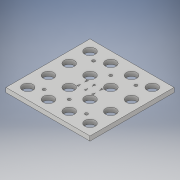
# Autodesk Inventor part: back_plate
Saved by Autodesk Inventor 2019 (Build 230136000, 136)
## iProperties
Created: 2019-08-25
Part Number: back_plate
Material: Generic
Document SubType Name: Modeling
Designer: Lino P
Density: 1 g/cm^3
Appearance: Default
Author: Lino P
Autodesk Inventor part; units mm, degrees
ref_plane "YZ Plane" through (0, 0, 0) normal (1, 0, 0) x (0, 1, 0)
ref_plane "XZ Plane" through (0, 0, 0) normal (0, 1, 0) x (-1, 0, 0)
ref_plane "XY Plane" through (0, 0, 0) normal (0, 0, 1) x (1, 0, 0)
sketch "Sketch1" plane through (0, 0, 0) normal (0, 1, 0) x (-1, 0, 0)
  line L0 (-85, 85) -> (85, 85)
  line L1 (85, 85) -> (85, -85)
  line L2 (85, -85) -> (-85, -85)
  line L3 (-85, -85) -> (-85, 85)
  line L4 (-85, 85) -> (85, -85) construction
  line L5 (85, 85) -> (-85, -85) construction
  point P0 (0, 0)
  point P1 (-63, -63)
  point P2 (-63, -21)
  point P3 (-63, 21)
  point P4 (-63, 63)
  point P5 (-21, -63)
  point P6 (-21, -21)
  point P7 (-21, 21)
  point P8 (-21, 63)
  point P9 (21, -63)
  point P10 (21, -21)
  point P11 (21, 21)
  point P12 (21, 63)
  point P13 (63, -63)
  point P14 (63, -21)
  point P15 (63, 21)
  point P16 (63, 63)
  dimension "d0" = 170
  dimension "d1" = 170
  dimension "d4" = 42
  dimension "d7" = 42
  constraints: 12 end point, 2 horizontal, 2 midpoint, 2 parallel, 1 perpendicular, 1 vertical, 15 other
  measures "d0" distance of L1.end L2.end
  measures "d1" distance of L0.end L1.end
  measures "d4" distance of point (-63, -63) point (-63, -21)
  measures "d7" distance of point (-63, -63) point (-21, -63)
extrude "Extrusion1" add sketch "Sketch1" along normal blind 9
hole "Hole1" at (63, 0, -63) at (63, 0, -21) at (63, 0, 21) at (63, 0, 63) at (21, 0, -63) at (21, 0, -21) at (21, 0, 21) at (21, 0, 63) at (-21, 0, -63) at (-21, 0, -21) at (-21, 0, 21) at (-21, 0, 63) at (-63, 0, -63) at (-63, 0, -21) at (-63, 0, 21) at (-63, 0, 63) direction (0, 1, 0) diameter 21 end through all both
sketch "Sketch2" plane through (0, 9, 0) normal (0, 1, 0) x (1, 0, 0)
  line L0 (-33.7, -4.15) -> (33.7, -4.15)
  line L1 (33.7, -4.15) -> (33.7, 4.15)
  line L2 (33.7, 4.15) -> (-33.7, 4.15)
  line L3 (-33.7, 4.15) -> (-33.7, -4.15)
  line L4 (-33.7, -4.15) -> (33.7, 4.15) construction
  line L5 (33.7, -4.15) -> (-33.7, 4.15) construction
  point P0 (0, 0)
  dimension "d19" = 67.4
  dimension "d20" = 8.3
  constraints: 12 end point, 2 midpoint, 2 parallel, 1 horizontal, 1 perpendicular
  measures "d19" distance of L2.end L1.end
  measures "d20" distance of L1.end L0.end
sketch "Sketch3" plane through (0, 9, 0) normal (0, 1, 0) x (1, 0, 0)
  line L0 (-42.7949, -50) -> (42.7949, -50) construction
  line L1 (42.7949, -50) -> (42.7949, 50) construction
  line L2 (42.7949, 50) -> (-42.7949, 50) construction
  line L3 (-42.7949, 50) -> (-42.7949, -50) construction
  line L4 (-42.7949, -50) -> (42.7949, 50) construction
  line L5 (42.7949, -50) -> (-42.7949, 50) construction
  point P0 (25, -42.5)
  point P1 (0, 0)
  dimension "d31" = 100
  constraints: 12 end point, 4 coincident, 2 midpoint, 2 parallel, 1 horizontal, 1 perpendicular
  measures "d31" distance of L1.end L0.end
hole "Hole3" at (-42.7949, 9, -50) at (42.7949, 9, -50) at (42.7949, 9, 50) at (-42.7949, 9, 50) direction (0, -1, 0) diameter 6 end through all both
sketch "Sketch4" plane through (0, 9, 0) normal (0, 1, 0) x (1, 0, 0)
  circle A0 centre (42.7949, -50) radius 3 construction
  circle A1 centre (-42.7949, 50) radius 3 construction
  circle A2 centre (42.7949, 50) radius 3 construction
  circle A3 centre (-42.7949, -50) radius 3 construction
  circle A4 centre (-63, -21) radius 10.5 construction
  circle A5 centre (-63, 63) radius 10.5 construction
  circle A6 centre (-21, -21) radius 10.5 construction
  circle A7 centre (-21, 63) radius 10.5 construction
  circle A8 centre (21, -21) radius 10.5 construction
  circle A9 centre (21, 63) radius 10.5 construction
  circle A10 centre (63, -21) radius 10.5 construction
  circle A11 centre (63, 63) radius 10.5 construction
  circle A12 centre (63, 21) radius 10.5 construction
  circle A13 centre (63, -63) radius 10.5 construction
  circle A14 centre (21, 21) radius 10.5 construction
  circle A15 centre (21, -63) radius 10.5 construction
  circle A16 centre (-21, 21) radius 10.5 construction
  circle A17 centre (-21, -63) radius 10.5 construction
  circle A18 centre (-63, 21) radius 10.5 construction
  circle A19 centre (-63, -63) radius 10.5 construction
  line L0 (-85, -85) -> (85, -85) construction
  line L1 (85, -85) -> (85, 85) construction
  line L2 (85, 85) -> (-85, 85) construction
  line L3 (-85, 85) -> (-85, -85) construction
  line L4 (-85, 85) -> (85, 85) construction
  line L5 (-7.5, -85) -> (7.5, -85) construction
  line L6 (7.5, -85) -> (7.5, 85) construction
  line L7 (7.5, 85) -> (-7.5, 85) construction
  line L8 (-7.5, 85) -> (-7.5, -85) construction
  line L9 (-7.5, -85) -> (7.5, 85) construction
  line L10 (7.5, -85) -> (-7.5, 85) construction
  line L11 (-21, 63) -> (21, 63) construction
  line L12 (21, 63) -> (21, 21) construction
  line L13 (21, 21) -> (-21, 21) construction
  line L14 (-21, 21) -> (-21, 63) construction
  line L15 (-85, 0) -> (85, 0) construction
  point P0 (0, 0)
  point P1 (0, 42)
  point P2 (0, -42)
  dimension "d39" = 15
  constraints: 22 end point, 4 midpoint, 4 parallel, 2 horizontal, 2 perpendicular, 1 point on line, 1 symmetric about line
  measures "d39" distance of L7.end L6.end
hole "Hole4" at (0, 9, -42) at (0, 9, 42) direction (0, -1, 0) diameter 6 end through all both
sketch "Sketch5" plane through (0, 9, 0) normal (0, 1, 0) x (1, 0, 0)
  line L0 (-33.7, -10) -> (33.7, -10) construction
  line L1 (33.7, -10) -> (33.7, 10) construction
  line L2 (33.7, 10) -> (-33.7, 10) construction
  line L3 (-33.7, 10) -> (-33.7, -10) construction
  line L4 (-33.7, -10) -> (33.7, 10) construction
  line L5 (33.7, -10) -> (-33.7, 10) construction
  line L6 (0, 10) -> (0, -10) construction
  line L7 (-1.8038, 10) -> (0, 4.1128)
  line L8 (1.8038, 10) -> (0, 4.1128)
  line L9 (-1.8038, 10) -> (1.8038, 10)
  line L10 (-33.7, 0) -> (33.7, 0) construction
  line L11 (-1.8038, -10) -> (0, -4.1128)
  line L12 (1.8038, -10) -> (0, -4.1128)
  line L13 (-1.8038, -10) -> (1.8038, -10)
  line L14 (-16.8038, 10) -> (-15, 4.1128)
  line L15 (-13.1962, 10) -> (-15, 4.1128)
  line L16 (-16.8038, 10) -> (-13.1962, 10)
  line L17 (13.1962, 10) -> (15, 4.1128)
  line L18 (16.8038, 10) -> (15, 4.1128)
  line L19 (13.1962, 10) -> (16.8038, 10)
  line L20 (-1.8038, 10) -> (0, 4.1128)
  line L21 (1.8038, 10) -> (0, 4.1128)
  line L22 (-1.8038, 10) -> (1.8038, 10)
  line L23 (-16.8038, -10) -> (-15, -4.1128)
  line L24 (-13.1962, -10) -> (-15, -4.1128)
  line L25 (-16.8038, -10) -> (-13.1962, -10)
  line L26 (13.1962, -10) -> (15, -4.1128)
  line L27 (16.8038, -10) -> (15, -4.1128)
  line L28 (13.1962, -10) -> (16.8038, -10)
  point P0 (0, 0)
  point P1 (-15, 10)
  point P2 (15, 10)
  point P3 (-15, -10)
  point P4 (15, -10)
  dimension "d47" = 67.4
  dimension "d50" = 20
  dimension "d53" = 15
  dimension "d56" = 15
  constraints: 58 end point, 12 symmetric about line, 6 midpoint, 3 horizontal, 2 parallel, 2 point on line, 1 collinear, 1 perpendicular, 21 other
  measures "d47" distance of L2.end L1.end
  measures "d50" distance between parallel lines of L0 L2
  measures "d53" distance of L6.start point (-15, 10)
  measures "d56" distance of L6.start point (15, 10)
extrude "Extrusion2" cut sketch "Sketch5" against normal blind 10 contours L9 L8 L7 | L11 L12 L13
extrude "Extrusion3" cut sketch "Sketch5" against normal blind 10 contours L16 L15 L14 | L19 L18 L17 | L23 L24 L25 | L26 L27 L28
body "Solid1"
